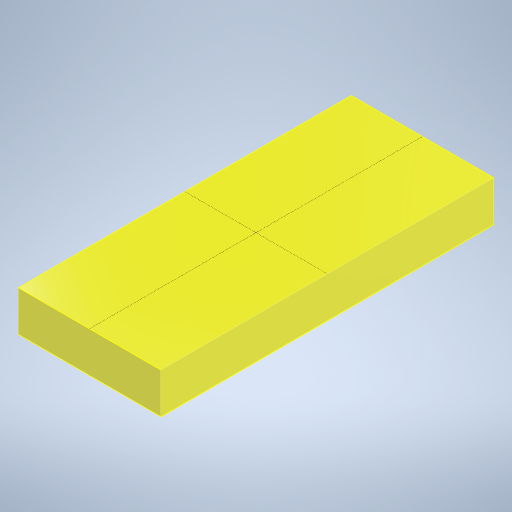
# Autodesk Inventor part: ball transfer unit base
Saved by Autodesk Inventor 2023 (Build 270158000, 158)
## iProperties
Created: 2022-12-06
Part Number: ball transfer unit base
Material: PLA Plastic
Document SubType Name: Modeling
Designer: mihal
Density: 1.25002 g/cm^3
Appearance: Yellow
Mass: 22.3129 g
Surface Area: 59 cm^2
Volume: 17.85 cm^3
Author: mihal
Autodesk Inventor part; units mm, degrees
ref_plane "YZ Plane" through (0, 0, 0) normal (1, 0, 0) x (0, 1, 0)
ref_plane "XZ Plane" through (0, 0, 0) normal (0, 1, 0) x (-1, 0, 0)
ref_plane "XY Plane" through (0, 0, 0) normal (0, 0, 1) x (1, 0, 0)
sketch "Sketch1" plane through (0, 0, 0) normal (0, 1, 0) x (-1, 0, 0)
  line L0 (0, 0) -> (30, 0)
  line L1 (30, 0) -> (30, -70)
  line L2 (30, -70) -> (0, -70)
  line L3 (0, -70) -> (0, 0)
  dimension "d0" = 30
  dimension "d1" = 70
  constraints: 8 end point, 2 parallel, 1 horizontal, 1 perpendicular
  measures "d0" distance of L1.end L2.end
  measures "d1" distance of L0.end L1.end
extrude "Extrusion1" add sketch "Sketch1" along normal blind 8.5
sketch "Sketch2" plane through (0, 8.5, 0) normal (0, 1, 0) x (1, 0, 0)
  line L0 (-30, 0) -> (0, 0) projected
  line L1 (-15, 0) -> (-15, 70) construction
  line L2 (0, 70) -> (-30, 70) projected
  line L3 (-30, 70) -> (-30, 0) projected
  line L4 (-30, 35) -> (0, 35) construction
  point P0 (-15, 35)
  constraints: 4 end point, 4 midpoint, 1 horizontal
sketch "Sketch3" plane through (0, 0, 0) normal (0, -1, 0) x (1, 0, 0)
  line L0 (0, -70) -> (-30, -70) projected
  line L1 (0, 0) -> (0, -70) projected
  line L2 (-30, 0) -> (0, 0) projected
  line L3 (-30, -70) -> (-30, 0) projected
  line L4 (-30, 0) -> (0, 0) projected
  line L5 (-15, 0) -> (-15, -70) construction
  line L6 (0, 0) -> (0, -70) projected
  line L7 (0, -35) -> (-30, -35) construction
  constraints: 4 end point, 4 midpoint
body "Solid1"
